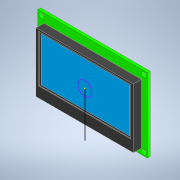
# Autodesk Inventor part: Adafruit_2675
Saved by Autodesk Inventor 2021 (Build 250183000, 183)
## iProperties
Created: 2020-11-05
Part Number: Adafruit_2675
Material: Generic
Document SubType Name: Modeling
Designer: Viktor
Density: 1 g/cm^3
Appearance: Default
Author: Viktor
Autodesk Inventor part; units mm, degrees
ref_plane "YZ Plane" through (0, 0, 0) normal (1, 0, 0) x (0, 1, 0)
ref_plane "XZ Plane" through (0, 0, 0) normal (0, 1, 0) x (-1, 0, 0)
ref_plane "XY Plane" through (0, 0, 0) normal (0, 0, 1) x (1, 0, 0)
sketch "Sketch1" plane through (0, 0, 0) normal (0, 0, 1) x (1, 0, 0)
  line L0 (-34, -23) -> (34, -23)
  line L1 (34, -23) -> (34, 23)
  line L2 (34, 23) -> (-34, 23)
  line L3 (-34, 23) -> (-34, -23)
  line L4 (-34, -23) -> (34, 23) construction
  line L5 (34, -23) -> (-34, 23) construction
  point P0 (0, 0)
  dimension "d0" = 68
  dimension "d1" = 46
  constraints: 12 end point, 2 midpoint, 2 parallel, 1 horizontal, 1 perpendicular
  measures "d0" distance of L1.end L2.end
  measures "d1" distance of L0.end L1.end
extrude "Extrusion1" add sketch "Sketch1" along normal blind 1.6
sketch "Sketch2" plane through (0, 0, 1.6) normal (0, 0, 1) x (1, 0, 0)
  line L0 (-47.6, 0) -> (47.6, 0) construction
  line L1 (0, -32.2) -> (0, 32.2) construction
  circle A0 centre (-31.8, 20.8) radius 1.6
  line L2 (34, 23) -> (-34, 23) construction
  line L3 (-34, 23) -> (-34, -23) construction
  circle A1 centre (31.8, 20.8) radius 1.6
  circle A2 centre (-31.8, -20.8) radius 1.6
  line L4 (34, -23) -> (-34, -23) construction
  circle A3 centre (31.8, -20.8) radius 1.6
  point P0 (0, 0)
  dimension "d4" = 3.2
  dimension "d5" = 0.6
  dimension "d6" = 0.6
  constraints: 4 centre point, 4 symmetric about line, 2 end point, 3 other
  measures "d4" diameter of A0
  measures "d5" distance edge to line of A0 L2
  measures "d6" distance edge to line of A0 L3
extrude "Extrusion2" cut sketch "Sketch2" against normal through all
sketch "Sketch3" plane through (0, 0, 1.6) normal (0, 0, 1) x (1, 0, 0)
  line L0 (0, 32.2) -> (0, -32.2) projected
  line L1 (-30.25, -19.5) -> (30.25, -19.5)
  line L2 (30.25, -19.5) -> (30.25, 17.5)
  line L3 (30.25, 17.5) -> (-30.25, 17.5)
  line L4 (-30.25, 17.5) -> (-30.25, -19.5)
  line L5 (-30.25, -19.5) -> (30.25, 17.5) construction
  line L6 (30.25, -19.5) -> (-30.25, 17.5) construction
  line L7 (-47.6, 0) -> (47.6, 0) projected
  point P0 (0, -1)
  dimension "d9" = 37
  dimension "d10" = 60.5
  dimension "d25" = 1
  constraints: 12 end point, 2 midpoint, 2 parallel, 1 horizontal, 1 perpendicular, 1 point on line
  measures "d9" distance of L3.end L1.start
  measures "d10" distance of L2.end L3.end
  measures "d25" distance from line of L7 point (0, -1)
extrude "Extrusion3" add sketch "Sketch3" along normal blind 5 separate body
sketch "Sketch4" plane through (0, 0, 6.6) normal (0, 0, 1) x (1, 0, 0)
  line L0 (0, -32.2) -> (0, 32.2) projected
  line L1 (-28.5, -12.99) -> (28.5, -12.99)
  line L2 (28.5, -12.99) -> (28.5, 16.5)
  line L3 (28.5, 16.5) -> (-28.5, 16.5)
  line L4 (-28.5, 16.5) -> (-28.5, -12.99)
  line L5 (-28.5, -12.99) -> (28.5, 16.5) construction
  line L6 (28.5, -12.99) -> (-28.5, 16.5) construction
  line L7 (30.25, 17.5) -> (-30.25, 17.5) projected
  point P0 (0, 0)
  point P1 (0, 1.755)
  dimension "d13" = 29.49
  dimension "d14" = 57
  dimension "d15" = 1
  constraints: 12 end point, 2 midpoint, 2 parallel, 1 horizontal, 1 perpendicular, 1 point on line
  measures "d13" distance of L3.end L1.start
  measures "d14" distance of L2.end L3.end
  measures "d15" distance between parallel lines of L7 L3
extrude "Extrusion4" cut sketch "Sketch4" against normal blind 0.5 bodies 2
sketch "Sketch5" plane through (0, 0, 6.1) normal (0, 0, 1) x (1, 0, 0)
  line L0 (0, 32.2) -> (0, -32.2) projected
  line L1 (-27.5, -12.07) -> (27.5, -12.07)
  line L2 (27.5, -12.07) -> (27.5, 15.42)
  line L3 (27.5, 15.42) -> (-27.5, 15.42)
  line L4 (-27.5, 15.42) -> (-27.5, -12.07)
  line L5 (-27.5, -12.07) -> (27.5, 15.42) construction
  line L6 (27.5, -12.07) -> (-27.5, 15.42) construction
  line L7 (30.25, 17.5) -> (-30.25, 17.5) projected
  point P0 (0, 0)
  point P1 (0, 1.675)
  dimension "d18" = 27.49
  dimension "d19" = 55
  dimension "d20" = 2.08
  constraints: 12 end point, 2 midpoint, 2 parallel, 1 horizontal, 1 perpendicular, 1 point on line
  measures "d18" distance of L3.end L1.start
  measures "d19" distance of L2.end L3.end
  measures "d20" distance between parallel lines of L7 L3
extrude "Extrusion5" cut sketch "Sketch5" against normal blind 0.5 bodies 2
sketch "Sketch6" plane through (0, 0, 5.6) normal (0, 0, 1) x (1, 0, 0)
  line L0 (27.5, -12.07) -> (-27.5, -12.07) projected
  line L1 (27.5, 15.42) -> (27.5, -12.07) projected
  line L2 (-27.5, 15.42) -> (27.5, 15.42) projected
  line L3 (-27.5, -12.07) -> (-27.5, 15.42) projected
  point P0 (0, 0)
extrude "Extrusion6" add sketch "Sketch6" along normal blind 0.5 separate body
sketch "Sketch7" plane through (0, 0, 6.6) normal (0, 0, 1) x (1, 0, 0)
  circle A0 centre (0, 0) radius 6.7082
  constraints: 1 centre point, 1 coincident
sketch "Sketch8" plane through (0, 0, 6.6) normal (0, 0, 1) x (1, 0, 0)
  circle A0 centre (0, 0) radius 4.3726
  line L0 (0, 0) -> (0, -28)
  constraints: 2 end point, 1 centre point, 1 coincident, 1 vertical
equation "\"d6\" = d5"
body "Solid1"
body "Solid2"
body "Solid3"
